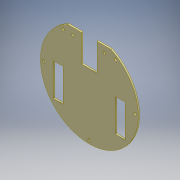
# Autodesk Inventor part: Tapa
Saved by Autodesk Inventor 2016 (Build 200138000, 138)
## iProperties
Created: 2019-03-15
Part Number: Tapa
Material: Nilón 6/6
Document SubType Name: Modeling
Designer: FIMCP
Mass: 34.0901 g
Surface Area: 318.751 cm^2
Volume: 30.1683 cm^3
Density: 1.13 g/cm^3
Appearance: Nilón 6
Author: FIMCP
Autodesk Inventor part; units mm, degrees
ref_plane "YZ Plane" through (0, 0, 0) normal (1, 0, 0) x (0, 1, 0)
ref_plane "XZ Plane" through (0, 0, 0) normal (0, 1, 0) x (-1, 0, 0)
ref_plane "XY Plane" through (0, 0, 0) normal (0, 0, 1) x (1, 0, 0)
sketch "Boceto1" plane through (0, 0, 0) normal (0, 1, 0) x (-1, 0, 0)
  arc A0 (-18, 72.808) -> (20, 72.2842) centre (0, 0) ccw
  line L0 (-18, 72.808) -> (-18, 72.2842)
  line L1 (55, 8) -> (40, 8)
  line L2 (40, 8) -> (40, -42)
  line L3 (40, -42) -> (55, -42)
  line L4 (55, -42) -> (55, 8)
  line L5 (-40, 8) -> (-55, 8)
  line L6 (-55, 8) -> (-55, -42)
  line L7 (-55, -42) -> (-40, -42)
  line L8 (-40, -42) -> (-40, 8)
  line L9 (20, 72.2842) -> (12, 72.2842)
  line L10 (12, 72.2842) -> (12, 25.2842)
  line L11 (-18, 72.808) -> (-12, 72.808)
  line L12 (-12, 72.808) -> (-12, 25.2842)
  line L13 (-18, 72.2842) -> (-18, 72.808)
  line L14 (12, 25.2842) -> (-12, 25.2842)
  line L15 (-30.8486, 25.2842) -> (-30.8486, 25)
  dimension "d0" = 150
  dimension "d1" = 18
  dimension "d3" = 15
  dimension "d4" = 50
  dimension "d5" = 15
  dimension "d6" = 50
  dimension "d7" = 40
  dimension "d8" = 40
  dimension "d28" = 24
  dimension "d29" = 12
  dimension "d33" = 8
  dimension "d34" = 8
  dimension "d36" = 47
  constraints: 32 end point, 5 horizontal, 5 parallel, 5 perpendicular, 2 point on circle, 1 centre point, 1 coincident, 1 point on line
  measures "d0" diameter of A0
  measures "d1" distance from line of L0 point (0, 0)
  measures "d3" distance of L3.end L3.start
  measures "d4" distance of L3.start L1.end
  measures "d5" distance of L8.start L7.start
  measures "d6" distance of L7.start L5.end
  measures "d7" distance from line of L8 point (0, 0)
  measures "d8" distance from line of L2 point (0, 0)
  measures "d28" distance between parallel lines of L12 L10
  measures "d29" distance from line of point (0, 0) L12
  measures "d33" distance from line of point (0, 0) L1
  measures "d34" distance from line of point (0, 0) L5
  measures "d36" distance between parallel lines of L14 L9
extrude "Extrusión1" add sketch "Boceto1" along normal blind 2
sketch "Boceto2" plane through (0, 0, 0) normal (0, 1, 0) x (-1, 0, 0)
  line L0 (-74.7999, 67.2842) -> (80.1068, 67.2842)
  line L1 (80.1068, 67.2842) -> (80.1068, 81.1614)
  line L2 (80.1068, 81.1614) -> (-74.7999, 81.1614)
  line L3 (-74.7999, 81.1614) -> (-74.7999, 67.2842)
  line L4 (20, 72.2842) -> (12, 72.2842) projected
  point P0 (0, 0)
  dimension "d13" = 5
  constraints: 8 end point, 2 parallel, 1 horizontal, 1 perpendicular
  measures "d13" distance between parallel lines of L4 L0
extrude "Extrusión2" cut sketch "Boceto2" along normal blind 2
sketch "Boceto3" plane through (0, 0, 0) normal (0, 1, 0) x (-1, 0, 0)
  circle A0 centre (-70, 0) radius 2
  circle A1 centre (0, -70) radius 2
  circle A2 centre (70, 0) radius 2
  point P0 (0, 0)
  dimension "d14" = 4
  dimension "d15" = 4
  dimension "d16" = 4
  dimension "d17" = 70
  dimension "d18" = 70
  dimension "d19" = 70
  constraints: 3 centre point
  measures "d14" diameter of A0
  measures "d15" diameter of A1
  measures "d16" diameter of A2
  measures "d17" distance of A0.centre point (0, 0)
  measures "d18" distance of A2.centre point (0, 0)
  measures "d19" distance of A1.centre point (0, 0)
extrude "Extrusión3" cut sketch "Boceto3" along normal mid plane 6
sketch "Boceto6" plane through (0, 0, 0) normal (0, 1, 0) x (-1, 0, 0)
  line L0 (-27, 57.2842) -> (-36.2309, 57.2842)
  arc A0 (-43.4373, 54.8927) -> (-36.2309, 57.2842) centre (-40.2309, 57.2842) ccw
  arc A1 (-27, 57.2842) -> (-23, 53.2842) centre (-23, 57.2842) ccw
  circle A2 centre (-23, 57.2842) radius 2
  arc A3 (25, 53.2842) -> (29, 57.2842) centre (25, 57.2842) ccw
  circle A4 centre (25, 57.2842) radius 2
  arc A5 (36.2309, 57.2842) -> (43.4373, 54.8927) centre (40.2309, 57.2842) ccw
  circle A6 centre (40.2309, 57.2842) radius 2
  circle A7 centre (-40.2309, 57.2842) radius 2
  point P0 (0, 0)
  dimension "d22" = 4
  dimension "d23" = 4
  dimension "d24" = 4
  dimension "d25" = 4
  constraints: 8 centre point, 8 point on circle, 4 coincident, 2 end point
  measures "d22" diameter of A2
  measures "d23" diameter of A4
  measures "d24" diameter of A6
  measures "d25" diameter of A7
extrude "Extrusión4" cut sketch "Boceto6" along normal mid plane 6
